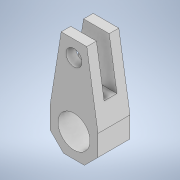
# Autodesk Inventor part: 11
Saved by Autodesk Inventor 2022 (Build 260153000, 153)
## iProperties
Created: 2022-03-14
Part Number: 11
Material: Všeobecné
Document SubType Name: Modeling
Designer: Šimon
Density: 1 g/cm^3
Appearance: Výchozí
Author: Šimon
Autodesk Inventor part; units mm, degrees
ref_plane "YZ Plane" through (0, 0, 0) normal (1, 0, 0) x (0, 1, 0)
ref_plane "XZ Plane" through (0, 0, 0) normal (0, 1, 0) x (-1, 0, 0)
ref_plane "XY Plane" through (0, 0, 0) normal (0, 0, 1) x (1, 0, 0)
sketch "Náčrt1" plane through (0, 0, 0) normal (0, 0, 1) x (1, 0, 0)
  line L0 (43, 17) -> (26, 0)
  line L1 (43, 17) -> (43, 43)
  line L2 (29, 130) -> (43, 43)
  line L3 (26, 0) -> (13, 0)
  line L4 (29, 130) -> (13, 130)
  line L5 (13, 134.5754) -> (13, -3.2687)
  line L6 (-17, 17) -> (0, 0)
  line L7 (-17, 17) -> (-17, 43)
  line L8 (-3, 130) -> (-17, 43)
  line L9 (0, 0) -> (13, 0)
  line L10 (-3, 130) -> (13, 130)
  dimension "d3" = 26
  dimension "d6" = 13
  dimension "d7" = 16
  constraints: 22 end point, 4 symmetric about line, 2 horizontal, 2 vertical
  measures "d3" distance of L0.start L1.end
  measures "d6" distance of L0.end L3.end
  measures "d7" distance of L2.start L4.end
extrude "Vysunutí1" add sketch "Náčrt1" along normal blind 40
sketch "Náčrt2" plane through (43, 17, 0) normal (1, 0, 0) x (0, 0, -1)
  line L0 (0, 113) -> (-40, 113) projected
  line L1 (-28, 113) -> (-28, 53)
  line L2 (-28, 53) -> (-12, 53)
  line L3 (-12, 53) -> (-12, 113)
  line L4 (-28, 113) -> (-12, 113)
  point P0 (0, -17)
  dimension "d10" = 60
  dimension "d11" = 16
  constraints: 8 end point, 3 perpendicular, 2 point on line, 1 vertical
  measures "d10" distance of L1.start L1.end
  measures "d11" distance of L1.end L2.end
extrude "Vysunutí2" cut sketch "Náčrt2" against normal through all
sketch "Náčrt3" plane through (0, 0, 40) normal (0, 0, 1) x (1, 0, 0)
  circle A0 centre (13, 30) radius 20
  circle A1 centre (13, 110) radius 10
  point P0 (0, 0)
  dimension "d14" = 40
  dimension "d15" = 20
  constraints: 2 centre point
  measures "d14" diameter of A0
  measures "d15" diameter of A1
extrude "Vysunutí3" cut sketch "Náčrt3" against normal through all contours A0
sketch "Náčrt4" plane through (0, 0, 40) normal (0, 0, 1) x (1, 0, 0)
  circle A0 centre (13, 110) radius 10
  point P0 (0, 0)
  dimension "d18" = 20
  constraints: 1 centre point
  measures "d18" diameter of A0
extrude "Vysunutí4" cut sketch "Náčrt4" against normal blind 20
